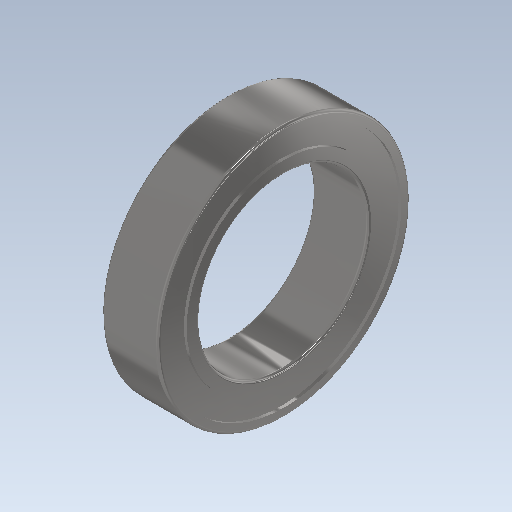
# Autodesk Inventor part: B6701ZZ
Saved by Autodesk Inventor 2021 (Build 250183000, 183)
## iProperties
Category: PARTsolutions
Company: MISUMI
Part Number: B6701ZZ
Material: 鉄、鋳鉄
Catalog Web Link: www.cadenas.de
Description: B6_ _ _ZZ, SB6_ _ _ZZ-Deep Groove Ball Bearings - Double Shield Type
Vendor: MISUMI
Document SubType Name: Modeling
Designer: partserver
Manufacturer: MISUMI
Mass: 3.83671 g
Surface Area: 6.81957 cm^2
Volume: 0.536603 cm^3
Density: 7.15 g/cm^3
Appearance: 鋼 - つや出し
PSOL_IDENT_0: {$CADENAS_DATA\23d-libs\misumi\metric\12_bearing_holders\sb6010zz.prj},171 {VTYP=3D},{NB=B6701ZZ},{L
PSOL_IDENT_1: INA=B6701ZZ},{NN=B6_ _ _ZZ, SB6_ _ _ZZ},{DATE=30.10.2020 16:03:36},{GEOMDATE=22.10.2019 06:26:04},{V
PSOL_IDENT_2: ERSION=},{LINEID=60},{WBVAR=TS},{WBNUMERIC=}  {NB=B6701ZZ},{LINA=B6701ZZ},{KT=DUMMY},{PN=B6701ZZ},{T
PSOL_IDENT_3: S=},{TS1= '', 'Steel', 'S', 'Stainless Steel'},{MAT=52100 Bearing Steel},{BN=6701ZZ},{DD=12},{D=18},
PSOL_IDENT_4: {B=4},{RR=0.2},{CR=0.92},{COR=0.53},{CRS=0.92},{CRSS=0.73},{CORS=0.53},{CORSS=0.42},{DD1=1.00},{R1=1
PSOL_IDENT_5: .00},{R2=1.0},{DSMIN=12.4},{DSMAX=13.86},{DS1=13.86},{DDHH=16.7},{R=0.2},{MASS=3},{MASS11=3},{AA=3.6
PSOL_IDENT_6: 000},{BB=0.6500},{CC=0.9300},{TYS=w/o Retaining Ring}
NB: B6701ZZ
NN: B6_ _ _ZZ, SB6_ _ _ZZ
NT: Deep Groove Ball Bearings - Double Shield Type
NBSYN: $PN.
LINA: B6701ZZ
CATALOG: Misumi
PN: B6701ZZ
TS: Steel
MAT: 52100 Bearing Steel
BN: 6701ZZ
DD: 12
D: 18
B: 4
RR: 0.2
CR: 0.92
COR: 0.53
DSMIN: 12.4
DSMAX: 13.86
DDHH: 16.7
R: 0.2
MASS: 3
SUPPLIER: MISUMI
ARTICLENO: B6701ZZ
BOMINFO: B6701ZZ
CREATOR: CADENAS GmbH
d1: 0.000 mm
Title: B6701ZZ
Author: Cadenas PARTsolutions
Comments: Deep Groove Ball Bearings - Double Shield Type
Autodesk Inventor part; units mm, degrees
sketch "Sketch_1" plane through (0, 0, 0) normal (0, 0, 1) x (1, 0, 0)
  line L0 (4, 0) -> (0, 0)
  arc A0 (0, 6.2) -> (0.2, 6) centre (0.2, 6.2) ccw
  line L1 (0.2, 6) -> (3.8, 6)
  arc A1 (3.8, 6) -> (4, 6.2) centre (3.8, 6.2) ccw
  line L2 (4, 6.2) -> (4, 6.93)
  line L3 (4, 6.93) -> (3.8, 6.93)
  line L4 (3.8, 6.93) -> (3.8, 8.35)
  line L5 (3.8, 8.35) -> (4, 8.35)
  line L6 (4, 8.35) -> (4, 8.8)
  arc A2 (4, 8.8) -> (3.8, 9) centre (3.8, 8.8) ccw
  line L7 (3.8, 9) -> (0.2, 9)
  arc A3 (0.2, 9) -> (0, 8.8) centre (0.2, 8.8) ccw
  line L8 (0, 8.8) -> (0, 8.35)
  line L9 (0, 8.35) -> (0.2, 8.35)
  line L10 (0.2, 8.35) -> (0.2, 6.93)
  line L11 (0.2, 6.93) -> (0, 6.93)
  line L12 (0, 6.93) -> (0, 6.2)
  constraints: 26 end point, 8 point on circle, 4 centre point
revolve "Revolution1" add sketch "Sketch_1" angle 360 about axis through (4, 0, 0) along (1, 0, 0)
ref_plane "center_point_XY" through (2, 0, 0) normal (1, 0, 0) x (0, 0, -1)
ref_plane "center_point_YZ" through (2, 0, 0) normal (0, 0, -1) x (0, 1, 0)
ref_plane "center_point_ZX" through (2, 0, 0) normal (0, 1, 0) x (1, 0, 0)
ref_plane "to_housing_XY" through (0, 0, 0) normal (1, 0, 0) x (0, 0, -1)
ref_plane "to_housing_YZ" through (0, 0, 0) normal (0, 0, -1) x (0, 1, 0)
ref_plane "to_housing_ZX" through (0, 0, 0) normal (0, 1, 0) x (1, 0, 0)
ref_plane "to_ring_XY" through (3.6, 0, 0) normal (1, 0, 0) x (0, 0, -1)
ref_plane "to_ring_YZ" through (3.6, 0, 0) normal (0, 0, -1) x (0, 1, 0)
ref_plane "to_ring_ZX" through (3.6, 0, 0) normal (0, 1, 0) x (1, 0, 0)
body "Solid1"
